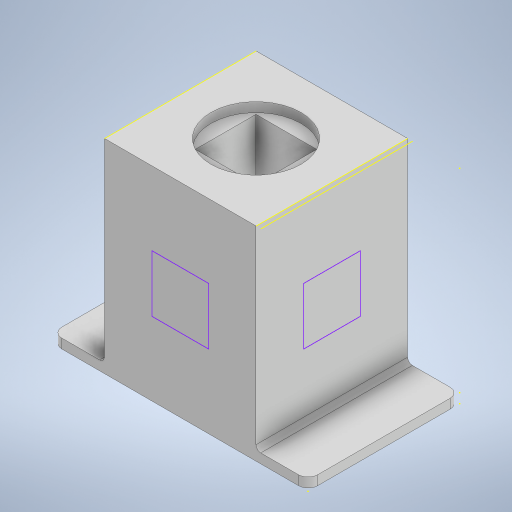
# Autodesk Inventor part: Cuvette Holder
Saved by Autodesk Inventor 2024 (Build 280153000, 153)
## iProperties
Created: 2023-06-23
Part Number: Cuvette Holder
Material: Generic
Document SubType Name: Modeling
Designer: Russe
Density: 1 g/cm^3
Appearance: Default
Author: Russe
Autodesk Inventor part; units mm, degrees
ref_plane "YZ Plane" through (0, 0, 0) normal (1, 0, 0) x (0, 1, 0)
ref_plane "XZ Plane" through (0, 0, 0) normal (0, 1, 0) x (-1, 0, 0)
ref_plane "XY Plane" through (0, 0, 0) normal (0, 0, 1) x (1, 0, 0)
sketch "Sketch1" plane through (0, 0, 0) normal (1, 0, 0) x (0, 1, 0)
  point P0 (0, 0)
sketch "Sketch2" plane through (0, 0, 0) normal (1, 0, 0) x (0, 1, 0)
  point P0 (0, 0)
sketch "Sketch3" plane through (0, 0, 0) normal (0, 1, 0) x (-1, 0, 0)
  point P0 (0, 0)
sketch "Sketch4" plane through (0, 0, 0) normal (0, 1, 0) x (-1, 0, 0)
  line L0 (52, 32) -> (2, 32)
  line L1 (0, 30) -> (0, 2)
  line L2 (2, 0) -> (52, 0)
  line L3 (54, 2) -> (54, 30)
  arc A0 (2, 32) -> (0, 30) centre (2, 30) ccw
  arc A1 (0, 2) -> (2, 0) centre (2, 2) ccw
  arc A2 (52, 0) -> (54, 2) centre (52, 2) ccw
  arc A3 (54, 30) -> (52, 32) centre (52, 30) ccw
  point P0 (0, 0)
  dimension "d0" = 2
  constraints: 8 end point, 8 point on circle, 8 tangent, 4 centre point, 3 equal radius, 2 parallel, 2 point on line, 1 horizontal, 1 perpendicular
  measures "d0" radius of A0
extrude "Extrusion1" add sketch "Sketch4" along normal blind 2
sketch "Sketch5" plane through (0, 2, 0) normal (0, 1, 0) x (1, 0, 0)
  point P0 (0, 0)
sketch "Sketch6" plane through (0, 2, 0) normal (0, 1, 0) x (1, 0, 0)
  point P0 (0, 0)
sketch "Sketch7" plane through (0, 2, 0) normal (0, 1, 0) x (1, 0, 0)
  line L0 (-11, 0) -> (-43, 0)
  line L1 (-43, 0) -> (-43, -32)
  line L2 (-43, -32) -> (-11, -32)
  line L3 (-11, -32) -> (-11, 0)
  point P0 (0, 0)
  constraints: 8 end point, 2 parallel, 1 horizontal, 1 perpendicular
extrude "Extrusion2" add sketch "Sketch7" along normal blind 41
fillet "Fillet1" radius 1 1 edges at (-11, 2, 16)
fillet "Fillet2" radius 1 1 edges at (-43, 2, 16)
sketch "Sketch8" plane through (-52, 0, 32) normal (0, 0, 1) x (1, 0, 0)
  point P0 (52, 0)
sketch "Sketch9" plane through (-52, 0, 32) normal (0, 0, 1) x (1, 0, 0)
  line L0 (19, 15.5) -> (31, 15.5)
  line L1 (31, 15.5) -> (31, 27.5)
  line L2 (31, 27.5) -> (19, 27.5)
  line L3 (19, 27.5) -> (19, 15.5)
  point P0 (52, 0)
  constraints: 8 end point, 2 parallel, 1 horizontal, 1 perpendicular
sketch "Sketch10" plane through (-11, 43, 32) normal (1, 0, 0) x (0, 0, -1)
  line L0 (10, -15.5) -> (22, -15.5)
  line L1 (22, -15.5) -> (22, -27.5)
  line L2 (22, -27.5) -> (10, -27.5)
  line L3 (10, -27.5) -> (10, -15.5)
  point P0 (32, -43)
  constraints: 8 end point, 2 parallel, 1 horizontal, 1 perpendicular
sketch "Sketch11" plane through (0, 43, 0) normal (0, 1, 0) x (1, 0, 0)
  line L0 (-43, -32) -> (-43, 0) projected
  line L1 (-11, 0) -> (-43, 0)
  line L2 (-2, 0) -> (-52, 0) projected
  circle A0 centre (-27, -16) radius 9.5
  point P0 (0, 0)
  constraints: 2 end point, 1 centre point, 1 point on line
sketch "Sketch12" plane through (0, 43, 0) normal (0, 1, 0) x (1, 0, 0)
  point P0 (0, 0)
sketch "Sketch13" plane through (0, 43, 0) normal (0, 1, 0) x (1, 0, 0)
  point P0 (0, 0)
extrude "Extrusion3" cut sketch "Sketch11" along normal blind 2
sketch "Sketch14" plane through (0, 43, 0) normal (0, 1, 0) x (1, 0, 0)
  line L0 (-43, 0) -> (-43, -32) projected
  line L1 (-11, -32) -> (-11, 0) projected
  line L2 (-10, -32) -> (-10, 0) projected
  point P0 (0, 0)
sketch "Sketch15" plane through (0, 43, 0) normal (0, 1, 0) x (1, 0, 0)
  line L0 (-20.6, -9.6) -> (-33.4, -9.6)
  line L1 (-33.4, -9.6) -> (-33.4, -22.4)
  line L2 (-33.4, -22.4) -> (-20.6, -22.4)
  line L3 (-20.6, -22.4) -> (-20.6, -9.6)
  point P0 (0, 0)
  constraints: 8 end point, 2 parallel, 1 horizontal, 1 perpendicular
sketch "Sketch16" plane through (0, 43, 0) normal (0, 1, 0) x (1, 0, 0)
  point P0 (0, 0)
sketch "Sketch17" plane through (0, 43, 0) normal (0, 1, 0) x (1, 0, 0)
  point P0 (0, 0)
extrude "Extrusion4" cut sketch "Sketch15" against normal blind 30
sketch "Sketch18" plane through (0, 43, 0) normal (0, 1, 0) x (1, 0, 0)
  point P0 (0, 0)
sketch "Sketch19" plane through (0, 43, 0) normal (0, 1, 0) x (1, 0, 0)
  circle A0 centre (-27, -16) radius 9.5
  point P0 (0, 0)
  constraints: 1 centre point
extrude "Extrusion5" cut sketch "Sketch19" against normal blind 2
body "Solid1"
